Autodesk Fusion 360 part; units mm, degrees
note: some values were not read from the file. Chosen so that the rebuilt part matches the saved one: which bodies a step acts on. Set by a fixed rule: which sketch regions a step uses.
(part 2 of 2)
sketch "Sketch33" plane through (0, 0, 0.2628) normal (0, 0, -1) x (1, 0, 0)
  circle A0 centre (90.2873, -26.9645) radius 2.5
  circle A1 centre (90.2873, -69.9645) radius 2.5
  line L0 (125, -25) -> (125, 0)
  line L1 (125, 0) -> (70.3336, 0)
  line L2 (70.3336, 0) -> (70.3336, -89.9645)
  line L3 (70.3336, -89.9645) -> (220.2873, -89.9645)
  line L4 (220.2873, -89.9645) -> (220.2873, 0.0355)
  line L5 (220.2873, 0.0355) -> (200.2873, 0.0355)
  line L6 (200.2873, 0.0355) -> (200.2873, 0)
  line L7 (200.2873, 0) -> (150.3104, 0)
  line L8 (150.3104, 0) -> (150.3104, -25)
  line L9 (150.3104, -25) -> (125, -25)
  circle A2 centre (136.2, -48.4645) radius 2
  circle A3 centre (200.2873, -69.9645) radius 2.5
  circle A4 centre (200.2873, -26.9645) radius 2.5
  line L10 (125, -25) -> (105, -25)
  line L11 (105, -25) -> (105, 0)
  constraint coincident L0.start L9.end
  constraint perpendicular L0 L10
  constraint perpendicular L9 L11
extrude "Extrude49" cut sketch "Sketch33" against normal blind 18 contours L0 L1 L10 L11 bodies 4
sketch "Sketch34" plane through (0, 0, 0) normal (0, 0, 1) x (1, 0, 0)
sketch "Sketch35" plane through (0, 0, -47.7372) normal (0, 0, -1) x (1, 0, 0)
  line L0 (142.4, -37.0645) -> (142.4, -59.8645)
  line L1 (142.4, -59.8645) -> (130, -59.8645)
  line L2 (130, -59.8645) -> (130, -37.0645)
  line L3 (130, -37.0645) -> (142.4, -37.0645)
  circle A0 centre (136.2, -62.8645) radius 1.5
  circle A1 centre (136.2, -34.0645) radius 1.5
  line L4 (146.4, -29.0645) -> (126, -29.0645)
  line L5 (126, -29.0645) -> (126, -67.8645)
  line L6 (126, -67.8645) -> (146.4, -67.8645)
  line L7 (146.4, -67.8645) -> (146.4, -29.0645)
  line L8 (-49.6, -20) -> (-49.6, -58.8)
  line L9 (-49.6, -58.8) -> (-70, -58.8)
  line L10 (-70, -58.8) -> (-70, -20)
  line L11 (-53.6, -50.8) -> (-66, -50.8)
  line L12 (-53.6, -44) -> (-53.6, -50.8)
  line L13 (-66, -44) -> (-66, -50.8)
  line L14 (-59.8, -41) -> (-56.3, -41)
  line L15 (-59.8, -41) -> (-63.3, -41)
  line L16 (-56.3, -19) -> (-63.3, -19)
  line L17 (-63.3, -19) -> (-63.3, -41)
  line L18 (-70, -20) -> (-66.3, -20)
  line L19 (-53.3, -20) -> (-49.6, -20)
  line L20 (-63.3, -19) -> (-63.3, -20)
  line L21 (-53.3, -19) -> (-53.3, -16)
  line L22 (-53.3, -16) -> (-53.3, -20)
  line L23 (-53.3, -16) -> (-67, -16)
  line L24 (-66.3, -19) -> (-66.3, -16)
  line L25 (-66.3, -19) -> (-66.3, -44)
  line L26 (-66.3, -44) -> (-53.3, -44)
  line L27 (-53.3, -20) -> (-53.3, -44)
  line L28 (-56.3, -19) -> (-56.3, -41)
  dimension "d215" = 20.4
  dimension "d216" = 38.8
  dimension "d224" = 3.5
  dimension "d225" = 3.5
  dimension "d226" = 22
  dimension "d227" = 7
  dimension "d228" = 3
  dimension "d229" = 3
  dimension "d230" = 3
  constraint horizontal L18
  constraint vertical L8
  constraint horizontal L9
  constraint vertical L10
  constraint perpendicular L10 L11
  constraint perpendicular L11 L12
  constraint perpendicular L11 L13
  constraint coincident L17 L20.end
  constraint collinear L18 L19
  constraint perpendicular L16 L20
  constraint parallel L12 L22
  constraint perpendicular L21 L23
  constraint coincident L23 L24.end
  constraint perpendicular L23 L24
  constraint perpendicular L22 L26
  constraint coincident L25 L18.end
  constraint coincident L26 L13.start
  constraint coincident L26 L12.start
  constraint perpendicular L26 L27
  constraint perpendicular L14 L28
  measures "d215" distance of L10.end L8.start
  measures "d216" distance of L10.end L9.end
  measures "d224" distance of L14.start L14.end
  measures "d225" distance of L14.start L15.end
  measures "d226" distance of L14.end L16.start
  measures "d227" distance of L16.start L16.end
  measures "d228" distance of L16.end L24.start
  measures "d229" distance of L16.start L21.start
  measures "d230" distance of L21.start L21.end
extrude "Extrude50" add sketch "Sketch35" along normal blind 7 separate body contours L21 L22 L23 L24 L25 L26 L27 makes body 5
sketch "Sketch36" plane through (0, 0, -54.7372) normal (0, 0, -1) x (1, 0, 0)
  line L0 (-63.3, -41) -> (-63.3, -19)
  line L1 (-63.3, -19) -> (-56.3, -19)
  line L2 (-56.3, -19) -> (-56.3, -41)
  line L3 (-56.3, -41) -> (-63.3, -41)
  line L4 (-53.3, -16) -> (-66.3, -16)
  line L5 (-66.3, -16) -> (-66.3, -44)
  line L6 (-66.3, -44) -> (-53.3, -44)
  line L7 (-53.3, -44) -> (-53.3, -16)
  line L8 (-66.3, -16) -> (-53.3, -16)
  line L9 (-53.3, -16) -> (-46.8, -16)
  line L10 (-66.3, -16) -> (-72.8, -16)
  line L11 (-72.8, -16) -> (-77.8, -16)
  line L12 (-46.8, -16) -> (-41.8, -16)
  line L13 (-46.8, -16) -> (-46.8, -44)
  line L14 (-46.8, -44) -> (-46.8, -49)
  line L15 (-72.8, -16) -> (-72.8, -44)
  line L16 (-72.8, -44) -> (-72.8, -49)
  line L17 (-72.8, -49) -> (-46.8, -49)
  line L18 (-72.8, -16) -> (-72.8, -11)
  line L19 (-72.8, -11) -> (-47, -11)
  line L20 (-47, -11) -> (-42, -11)
  line L21 (-42, -11) -> (-42, -49)
  line L22 (-42, -49) -> (-46.8, -49)
  line L23 (-72.8, -49) -> (-77.8, -49)
  line L24 (-77.8, -49) -> (-77.8, -11)
  line L25 (-77.8, -11) -> (-72.8, -11)
  line L26 (-77.8, -11) -> (-77.8, -6)
  line L27 (-42, -11) -> (-42, -6)
  dimension "d233" = 6.5
  dimension "d234" = 6.5
  dimension "d235" = 5
  dimension "d236" = 5
  dimension "d237" = 5
  dimension "d238" = 5
  dimension "d239" = 5
  dimension "d240" = 5
  dimension "d241" = 5
  dimension "d242" = 5
  constraint coincident L4.end L5.start
  constraint coincident L4.start L7.end
  constraint perpendicular L7 L9
  constraint perpendicular L5 L10
  constraint perpendicular L0 L11
  constraint perpendicular L7 L12
  constraint perpendicular L9 L13
  constraint perpendicular L9 L14
  constraint perpendicular L11 L15
  constraint perpendicular L11 L16
  constraint perpendicular L14 L17
  constraint perpendicular L10 L18
  constraint perpendicular L18 L19
  constraint perpendicular L18 L20
  constraint perpendicular L20 L21
  constraint perpendicular L16 L23
  constraint perpendicular L11 L24
  constraint perpendicular L25 L26
  constraint perpendicular L20 L27
  measures "d233" distance of L4.start L9.end
  measures "d234" distance of L4.end L10.end
  measures "d235" distance of L10.end L11.end
  measures "d236" distance of L9.end L12.end
  measures "d237" distance of L13.end L14.end
  measures "d238" distance of L15.end L16.end
  measures "d239" distance of L10.end L18.end
  measures "d240" distance of L16.end L23.end
  measures "d241" distance of L24.end L26.end
  measures "d242" distance of L20.end L27.end
extrude "Extrude51" add sketch "Sketch36" along normal blind 5 contours L0 L1 L2 L3 | L4 L5 L6 L7 L8 | L5 L6 L7 L9 L10 L13 L14 L15 L16 L17 | L4 L8 L9 L10 L12 L18 L19 L20 L21 | L12 L13 L14 L21 L22 | L11 L15 L16 L23 L24 | L11 L18 L24 L25 bodies 5
extrude "Extrude52" cut 1 faces at (-65.8, 36.3333, -59.7372) along direction (0, 0, 1) blind 2 on bodies 5 bodies 5
sketch "Sketch37" plane through (0, 0, -57.7372) normal (0, 0, -1) x (1, 0, 0)
  line L0 (-77.8, -49) -> (-46.8, -49)
  line L1 (-46.8, -49) -> (-42, -49)
  line L2 (-42, -49) -> (-42, -11)
  line L3 (-42, -11) -> (-72.8, -11)
  line L4 (-72.8, -11) -> (-77.8, -11)
  line L5 (-77.8, -11) -> (-77.8, -49)
  line L6 (-77.8, -11) -> (-72.8, -11)
  line L7 (-72.8, -11) -> (-72.8, -49)
  line L8 (-42, -11) -> (-47, -11)
  line L9 (-47, -11) -> (-46.8, -49)
  dimension "d247" = 5
  dimension "d248" = 5
  constraint coincident L4.end L5.start
  constraint perpendicular L5 L6
  constraint coincident L0 L7.end
  constraint perpendicular L0 L7
  constraint coincident L2.end L3.start
  constraint perpendicular L2 L8
  constraint coincident L0.end L1.start
  measures "d247" distance of L4.end L3.end
  measures "d248" distance of L2.end L8.end
extrude "Extrude53" add sketch "Sketch37" along normal blind 30 contours L0 L4 L5 L6 L7 | L1 L2 L3 L8 L9 bodies 5
sketch "Sketch38" plane through (0, 0, -57.7372) normal (0, 0, -1) x (1, 0, 0)
  line L0 (-46.8, -49) -> (-47, -11)
  line L1 (-47, -11) -> (-72.8, -11)
  line L2 (-72.8, -11) -> (-72.8, -49)
  line L3 (-72.8, -49) -> (-46.8, -49)
  line L4 (-59.9, -11) -> (-59.9, -16)
  line L5 (-59.9, -16) -> (-72.8, -16)
  line L6 (-59.9, -16) -> (-46.974, -15.932)
  dimension "d251" = 5
  constraint midpoint L1 L4.start
  constraint perpendicular L1 L4
  constraint coincident L2 L5.end
  constraint perpendicular L2 L5
  constraint coincident L0 L6.end
  constraint perpendicular L0 L6
  measures "d251" distance of L4.start L4.end
extrude "Extrude54" add sketch "Sketch38" along normal blind 30 contours L0 L1 L4 L6 | L1 L2 L4 L5 bodies 5
sketch "Sketch39" plane through (0, 0, -57.7372) normal (0, 0, -1) x (1, 0, 0)
  line L0 (-59.9, -16) -> (-72.8, -16)
  line L1 (-72.8, -16) -> (-72.8, -49)
  line L2 (-72.8, -49) -> (-46.8, -49)
  line L3 (-46.8, -49) -> (-46.974, -15.932)
  line L4 (-46.974, -15.932) -> (-59.9, -16)
extrude "Extrude55" add 1 faces at (-77.8, 36.3333, -65.7372) along direction (-1, 0, 0) blind 2.5 on bodies 5 bodies 5
extrude "Extrude56" cut 1 faces at (-72.8, 27, -77.7372) along direction (-1, 0, 0) blind 2.5 on bodies 5 bodies 5
extrude "Extrude57" add 1 faces at (-42, 36.3333, -65.7372) along direction (1, 0, 0) blind 2.5 on bodies 5 bodies 5
extrude "Extrude58" cut 1 faces at (-46.916, 26.9546, -77.7372) along direction (0.999986, -0.005263, 0) blind 2.5 on bodies 5 bodies 5
delete_face "DeleteFace1" 1 faces at (-43.6, 49, -66.7372) on bodies 5
extrude "Extrude59" add 1 faces at (-45.9667, 48.9956, -77.7372) along direction (-0.005263, -0.999986, 0) blind 5 on bodies 5 bodies 5
sketch "Sketch40" plane through (0, 0, -87.7372) normal (0, 0, -1) x (1, 0, 0)
  line L0 (-46.8, -49) -> (-39.5, -49)
  line L1 (-39.5, -49) -> (-39.5, -11)
  line L2 (-39.5, -11) -> (-80.3, -11)
  line L3 (-80.3, -11) -> (-80.3, -49)
  line L4 (-80.3, -49) -> (-75.3, -49)
  line L5 (-75.3, -49) -> (-75.3, -16)
  line L6 (-75.3, -16) -> (-59.9, -16)
  line L7 (-59.9, -16) -> (-44.4741, -15.9188)
  line L8 (-44.4741, -15.9188) -> (-44.3264, -43.9869)
  line L9 (-44.3264, -43.9869) -> (-46.8263, -44.0001)
  line L10 (-46.8263, -44.0001) -> (-46.8, -49)
  line L11 (-44.3264, -43.9869) -> (-44.3264, -49)
  constraint coincident L8.end L9.start
  constraint coincident L0 L11.end
  constraint perpendicular L0 L11
extrude "Extrude60" cut sketch "Sketch40" against normal blind 30 contours L0 L9 L10 L11 bodies 5
sketch "Sketch41" plane through (0, 0, -6.7372) normal (0, 0, -1) x (1, 0, 0)
  circle A0 centre (136.2, -48.4645) radius 2
  line L0 (142.4, -59.3645) -> (146.4, -59.3645)
  line L1 (146.4, -59.3645) -> (146.4, -37.3645)
  line L2 (146.4, -37.3645) -> (142.4, -37.3645)
  line L3 (142.4, -37.3645) -> (142.4, -37.0645)
  line L4 (142.4, -37.0645) -> (130, -37.0645)
  line L5 (130, -37.0645) -> (130, -37.3645)
  line L6 (130, -37.3645) -> (126, -37.3645)
  line L7 (126, -37.3645) -> (126, -59.3645)
  line L8 (126, -59.3645) -> (130, -59.3645)
  line L9 (130, -59.3645) -> (130, -59.8645)
  line L10 (130, -59.8645) -> (142.4, -59.8645)
  line L11 (142.4, -59.8645) -> (142.4, -59.3645)
  line L12 (136.2, -48.4645) -> (136.2, -25)
  line L13 (136.2, -25) -> (136.2, -31)
  line L14 (136.2, -25) -> (136.2, -31)
  line L15 (136.2, -31) -> (136.2, -15)
  line L16 (136.2, -15) -> (136.2, -12)
  line L17 (136.2, -12) -> (146, -12)
  line L18 (146, -12) -> (128, -12)
  dimension "d266" = 6
  dimension "d267" = 6
  dimension "d268" = 16
  dimension "d269" = 3
  constraint coincident A0.centre L12.start
  constraint perpendicular L4 L12
  constraint perpendicular L4 L13
  constraint perpendicular L4 L14
  constraint parallel L12 L15
  constraint parallel L15 L16
  constraint perpendicular L16 L17
  constraint parallel L17 L18
  measures "d266" distance of L12.end L13.end
  measures "d267" distance of L12.end L13.end
  measures "d268" distance of L13.end L15.end
  measures "d269" distance of L15.end L16.end
sketch "Sketch42" plane through (0, 0, -54.7372) normal (0, 0, 1) x (-1, 0, 0)
  line L0 (53.3, -44) -> (53.3, -16)
  line L1 (53.3, -16) -> (66.3, -16)
  line L2 (66.3, -16) -> (66.3, -44)
  line L3 (66.3, -44) -> (53.3, -44)
  line L4 (39.5, -49) -> (80.3, -49)
  line L5 (80.3, -49) -> (80.3, -11)
  line L6 (80.3, -11) -> (77.8, -11)
  line L7 (77.8, -11) -> (72.8, -11)
  line L8 (72.8, -11) -> (39.5, -11)
  line L9 (39.5, -11) -> (39.5, -49)
sketch "Sketch43" plane through (0, 0, -57.7372) normal (0, 0, -1) x (1, 0, 0)
  line L0 (-60, -49) -> (-60, -44)
  dimension "d270" = 5
  constraint vertical L0
  measures "d270" distance of L0.start L0.end
sketch "Sketch44" plane through (0, 49, 0) normal (0, 1, 0) x (-1, 0, 0)
  line L0 (44.3264, -57.7372) -> (75.3, -57.7372)
  line L1 (75.3, -57.7372) -> (75.3, -87.7372)
  line L2 (75.3, -87.7372) -> (80.3, -87.7372)
  line L3 (80.3, -87.7372) -> (80.3, -54.7372)
  line L4 (80.3, -54.7372) -> (39.5, -54.7372)
  line L5 (39.5, -54.7372) -> (39.5, -87.7372)
  line L6 (39.5, -87.7372) -> (44.3264, -87.7372)
  line L7 (44.3264, -87.7372) -> (44.3264, -57.7372)
extrude "Extrude61" add sketch "Sketch44" along normal blind 8 bodies 5
extrude "Extrude62" cut 1 faces at (-78.6333, 57, -66.7372) along direction (0, -1, 0) blind 13 on bodies 5 bodies 5
sketch "Sketch45" plane through (0, 44, 0) normal (0, 1, 0) x (-1, 0, 0)
  line L0 (66.3, -47.7372) -> (53.3, -47.7372)
  line L1 (53.3, -47.7372) -> (53.3, -54.7372)
  line L2 (53.3, -54.7372) -> (39.5, -54.7372)
  line L3 (39.5, -54.7372) -> (39.5, -87.7372)
  line L4 (39.5, -87.7372) -> (44.3264, -87.7372)
  line L5 (44.3264, -87.7372) -> (44.3264, -57.7372)
  line L6 (44.3264, -57.7372) -> (75.3, -57.7372)
  line L7 (75.3, -57.7372) -> (75.3, -87.7372)
  line L8 (75.3, -87.7372) -> (80.3, -87.7372)
  line L9 (80.3, -87.7372) -> (80.3, -54.7372)
  line L10 (80.3, -54.7372) -> (66.3, -54.7372)
  line L11 (66.3, -54.7372) -> (66.3, -47.7372)
  line L12 (44.3264, -57.7372) -> (44.3264, -54.7372)
  line L13 (75.3, -57.7372) -> (75.3, -54.7372)
  constraint coincident L5.end L6.start
  constraint coincident L2 L12.end
  constraint perpendicular L2 L12
  constraint coincident L6.end L7.start
  constraint coincident L10 L13.end
  constraint perpendicular L10 L13
extrude "Extrude63" add sketch "Sketch45" along normal blind 30 contours L7 L8 L9 L10 L13 | L2 L3 L4 L5 L12 bodies 5
extrude "Extrude64" add 2 faces at (-41.1088, 74, -65.7372) (-76.9667, 74, -65.7372) along direction (0, 1, 0) blind 10 on bodies 5 bodies 5
extrude "Extrude65" add 1 faces at (-59.8421, 34.6623, -57.7372) along direction (0, 0, -1) blind 30 on bodies 5 bodies 5
extrude "Extrude66" add 2 faces at (-41.1088, 84, -65.7372) (-76.9667, 84, -65.7372) along direction (0, 1, 0) blind 5 on bodies 5 bodies 5
sketch "Sketch46" plane through (-80.3, 0, 0) normal (-1, 0, 0) x (0, -1, 0)
  line L0 (-89, -87.7372) -> (-11, -87.7372)
  line L1 (-11, -87.7372) -> (-11, -54.7372)
  line L2 (-11, -54.7372) -> (-89, -54.7372)
  line L3 (-89, -54.7372) -> (-89, -87.7372)
  line L4 (-89, -65.3059) -> (-81, -65.3059)
  line L5 (-89, -54.7372) -> (-89, -62.7372)
  line L6 (-89, -62.7372) -> (-81, -62.7372)
  line L7 (-81, -62.7372) -> (-81, -57.7372)
  line L8 (-81, -65.3059) -> (-64, -65.3059)
  line L9 (-81, -62.7372) -> (-64, -62.7372)
  line L10 (-81, -65.3059) -> (-81, -57.3059)
  line L11 (-81, -57.3059) -> (-64, -57.3059)
  line L12 (-64, -57.3059) -> (-64, -65.3059)
  dimension "d283" = 8
  dimension "d284" = 8
  dimension "d285" = 8
  dimension "d286" = 5
  dimension "d287" = 17
  dimension "d288" = 17
  dimension "d289" = 8
  constraint coincident L3 L4.start
  constraint perpendicular L3 L4
  constraint coincident L2.end L3.start
  constraint perpendicular L4 L5
  constraint perpendicular L5 L6
  constraint perpendicular L4 L7
  constraint perpendicular L3 L8
  constraint perpendicular L7 L9
  constraint perpendicular L6 L10
  constraint perpendicular L10 L11
  measures "d283" distance of L4.start L4.end
  measures "d284" distance of L2.end L5.end
  measures "d285" distance of L5.end L6.end
  measures "d286" distance of L6.end L7.end
  measures "d287" distance of L4.end L8.end
  measures "d288" distance of L6.end L9.end
  measures "d289" distance of L4.end L10.end
extrude "Extrude67" add sketch "Sketch46" along normal blind 13 contours L8 L9 L10 L12 | L7 L9 L10 L11 L12 bodies 5
sketch "Sketch47" plane through (0, 81, 0) normal (0, 1, 0) x (-1, 0, 0)
  line L0 (80.3, -57.3059) -> (80.3, -65.3059)
  line L1 (80.3, -65.3059) -> (93.3, -65.3059)
  line L2 (93.3, -65.3059) -> (93.3, -57.3059)
  line L3 (93.3, -57.3059) -> (80.3, -57.3059)
  line L4 (80.3, -65.3059) -> (86.3, -65.3059)
  line L5 (86.3, -65.3059) -> (86.3, -62.3059)
  circle A0 centre (86.3, -62.3059) radius 1.5
  dimension "d292" = 6
  dimension "d293" = 3
  dimension "d294" = 3
  constraint coincident L0.end L1.start
  constraint perpendicular L0 L4
  constraint perpendicular L4 L5
  constraint coincident L5.end A0.centre
  measures "d292" distance of L0.end L4.end
  measures "d293" distance of L4.end L5.end
  measures "d294" diameter of A0
extrude "Extrude68" cut sketch "Sketch47" against normal blind 13 contours A0 bodies 5
extrude "Extrude69" cut 1 faces at (-88.9667, 75.3333, -57.3059) along direction (0, 0, -1) blind 2 on bodies 5 bodies 5
extrude "Extrude70" add 1 faces at (-52.2088, 22, -87.7372) along direction (0, 0, -1) blind 5 on bodies 5 bodies 5
sketch "Sketch48" plane through (0, 89, 0) normal (0, 1, 0) x (-1, 0, 0)
  line L0 (80.3, -92.7372) -> (80.3, -54.7372)
  line L1 (80.3, -54.7372) -> (75.3, -54.7372)
  line L2 (75.3, -54.7372) -> (75.3, -92.7372)
  line L3 (75.3, -92.7372) -> (80.3, -92.7372)
sketch "Sketch49" plane through (-80.3, 0, 0) normal (-1, 0, 0) x (0, -1, 0)
  line L0 (-81, -65.3059) -> (-81, -59.3059)
  line L1 (-81, -59.3059) -> (-64, -59.3059)
  line L2 (-64, -59.3059) -> (-64, -65.3059)
  line L3 (-64, -65.3059) -> (-81, -65.3059)
  line L4 (-11, -92.7372) -> (-11, -54.7372)
  line L5 (-11, -54.7372) -> (-89, -54.7372)
  line L6 (-89, -54.7372) -> (-89, -92.7372)
  line L7 (-89, -92.7372) -> (-11, -92.7372)
sketch "Sketch50" plane through (0, 89, 0) normal (0, 1, 0) x (-1, 0, 0)
sketch "Sketch51" plane through (-80.3, 0, 0) normal (-1, 0, 0) x (0, -1, 0)
sketch "Sketch52" plane through (0, 0, 0) normal (0, 1, 0) x (1, 0, 0)
  line L0 (-10, -20) -> (-50.8, -20)
  line L1 (-50.8, -20) -> (-50.8, -58)
  line L2 (-50.8, -58) -> (-50.8, -49)
  line L3 (-53.3, -49) -> (-56.8, -49)
  line L4 (-56.8, -49) -> (-60.3, -49)
  line L5 (-56.8, -49) -> (-53.3, -49)
  line L6 (-56.8, -49) -> (-60.3, -49)
  line L7 (-53.3, -49) -> (-53.3, -65)
  line L8 (-60.3, -49) -> (-60.3, -65)
  line L9 (-60.3, -65) -> (-53.3, -65)
  line L10 (-82, -49) -> (-82, -46)
  line L11 (-63.3, -46) -> (-50.8, -46)
  line L12 (-63.3, -68) -> (-50.8, -68)
  line L13 (-50.8, -68) -> (-50.8, -58)
  line L14 (-72.8, 54.7372) -> (-39.5, 54.7372)
  line L15 (-39.5, 92.7372) -> (-80.3, 92.7372)
  line L16 (-60.3, -49) -> (-63.3, -49)
  line L17 (-63.3, -49) -> (-63.3, -68)
  line L18 (-63.3, -49) -> (-63.3, -46)
  line L19 (-50.8, -68) -> (-10, -68)
  line L20 (-10, -20) -> (-10, -68)
  dimension "d301" = 38
  dimension "d302" = 9
  dimension "d303" = 6
  dimension "d305" = 3.5
  dimension "d306" = 3.5
  dimension "d307" = 16
  dimension "d308" = 16
  dimension "d311" = 3
  dimension "d312" = 33.3
  dimension "d313" = 40.8
  dimension "d314" = 40.8
  dimension "d315" = 3
  constraint horizontal L0
  constraint perpendicular L0 L1
  constraint parallel L1 L2
  constraint perpendicular L2 L3
  constraint parallel L3 L4
  constraint parallel L3 L5
  constraint perpendicular L2 L6
  constraint perpendicular L5 L7
  constraint perpendicular L4 L8
  constraint coincident L1 L11.end
  constraint perpendicular L1 L11
  constraint perpendicular L9 L13
  constraint perpendicular L8 L16
  constraint perpendicular L12 L17
  constraint perpendicular L11 L18
  constraint perpendicular L13 L19
  constraint perpendicular L19 L20
  measures "d301" distance of L0.end L1.end
  measures "d302" distance of L1.end L2.end
  measures "d303" distance of L2.end L3.end
  measures "d305" distance of L3.end L3.start
  measures "d306" distance of L3.end L4.end
  measures "d307" distance of L3.start L7.end
  measures "d308" distance of L4.end L8.end
  measures "d311" distance of L10.start L10.end
  measures "d312" distance of L14.start L14.end
  measures "d313" distance of L15.start L15.end
  measures "d314" distance of L0.start L0.end
  measures "d315" distance of L4.end L16.end
extrude "Extrude71" add sketch "Sketch52" along normal blind 5 separate body makes body 6
sketch "Sketch53" plane through (0, 5, 0) normal (0, 1, 0) x (-1, 0, 0)
  line L0 (60.3, 49) -> (53.3, 49)
  line L1 (53.3, 49) -> (53.3, 65)
  line L2 (53.3, 65) -> (60.3, 65)
  line L3 (60.3, 65) -> (60.3, 49)
  line L4 (50.8, 20) -> (50.8, 46)
  line L5 (50.8, 46) -> (63.3, 46)
  line L6 (63.3, 46) -> (63.3, 68)
  line L7 (63.3, 68) -> (10, 68)
  line L8 (10, 68) -> (10, 20)
  line L9 (10, 20) -> (50.8, 20)
  line L10 (53.3, 65) -> (60.3, 65)
  line L11 (60.3, 65) -> (60.3, 49)
  line L12 (60.3, 49) -> (53.3, 49)
  line L13 (53.3, 49) -> (53.3, 65)
  constraint horizontal L10
  constraint vertical L11
  constraint horizontal L12
  constraint vertical L13
  constraint coincident L0.start L3.end
  constraint coincident L1.end L2.start
extrude "Extrude72" add sketch "Sketch53" against normal blind 2 contours L0 L1 L2 L3 L10 L11 L12 L13 bodies 6
move_body "Move3" bodies 6 to x (1, 0, 0) y (0, 1, 0) z (0, 0, 1) at (-31.7357, 93.4456, -113.0049)
sketch "Sketch54" plane through (150.2873, 0, 0) normal (-1, 0, 0) x (0, -1, 0)
  line L0 (-25, 7.2628) -> (-25, 18.2628)
  line L1 (-25, 18.2628) -> (-21.9645, 18.2628)
  line L2 (-21.9645, 18.2628) -> (-21.9645, 50.4628)
  line L3 (-21.9645, 50.4628) -> (-69.9645, 50.4628)
  line L4 (-69.9645, 50.4628) -> (-69.9645, 7.2628)
  line L5 (-69.9645, 7.2628) -> (-25, 7.2628)
  circle A0 centre (-64.3645, 12.8628) radius 1.5
  circle A1 centre (-64.3645, 44.8628) radius 1.5
  circle A2 centre (-32.5645, 12.8628) radius 1.5
  circle A3 centre (-32.5645, 44.8628) radius 1.5
  circle A4 centre (-48.4645, 28.8628) radius 11.5
  line L6 (-48.4645, 28.8628) -> (-21.9645, 28.8628)
  constraint coincident A4.centre L6.start
  constraint coincident L2 L6.end
  constraint perpendicular L2 L6
sketch "Sketch55" plane through (150.2873, 0, 0) normal (-1, 0, 0) x (0, -1, 0)
  line L0 (-150, 30) -> (-180, 30)
  line L1 (-180, 30) -> (-180, 35)
  line L2 (-180, 30) -> (-180, 25)
  line L3 (-180, 35) -> (-150, 35)
  line L4 (-150, 35) -> (-150, 25)
  line L5 (-150, 25) -> (-180, 25)
  line L6 (-150, 35) -> (-140, 35)
  line L7 (-140, 35) -> (-140, -65)
  line L8 (-150, 25) -> (-150, -65)
  line L9 (-150, -65) -> (-140, -65)
  dimension "d320" = 30
  dimension "d321" = 5
  dimension "d322" = 5
  dimension "d323" = 10
  dimension "d324" = 100
  dimension "d325" = 90
  constraint horizontal L0
  constraint perpendicular L0 L1
  constraint perpendicular L0 L2
  constraint perpendicular L1 L3
  constraint perpendicular L0 L4
  constraint perpendicular L2 L5
  constraint perpendicular L4 L6
  constraint perpendicular L6 L7
  constraint perpendicular L5 L8
  measures "d320" distance of L0.start L0.end
  measures "d321" distance of L0.end L1.end
  measures "d322" distance of L0.end L2.end
  measures "d323" distance of L3.end L6.end
  measures "d324" distance of L6.end L7.end
  measures "d325" distance of L4.end L8.end
extrude "Extrude73" add sketch "Sketch55" along normal blind 10 separate body makes body 7
sketch "Sketch56" plane through (0, 0, -65) normal (0, 0, -1) x (1, 0, 0)
  line L0 (150.2873, -150) -> (150.2873, -140)
  line L1 (150.2873, -140) -> (140.2873, -140)
  line L2 (140.2873, -140) -> (140.2873, -150)
  line L3 (140.2873, -150) -> (150.2873, -150)
  line L4 (140.2873, -150) -> (145.2873, -150)
  line L5 (145.2873, -150) -> (145.2873, -145)
  circle A0 centre (145.2873, -145) radius 5
  dimension "d328" = 5
  dimension "d329" = 5
  dimension "d330" = 10
  constraint coincident L2.end L3.start
  constraint perpendicular L2 L4
  constraint perpendicular L4 L5
  constraint coincident L5.end A0.centre
  measures "d328" distance of L2.end L4.end
  measures "d329" distance of L4.end L5.end
  measures "d330" diameter of A0
extrude "Extrude74" cut sketch "Sketch56" against normal blind 90 contours L0 L3 A0 | L0 L1 A0 | L2 L3 L4 A0 | L1 L2 A0 bodies 7
extrude "Extrude75" add 1 faces at (146.954, 180, 31.6667) along direction (0, 1, 0) blind 8 on bodies 7 bodies 7
sketch "Sketch57" plane through (140.2873, 0, 0) normal (-1, 0, 0) x (0, -1, 0)
  line L0 (-188, 25) -> (-145, 25)
  line L1 (-145, 25) -> (-140, 25)
  line L2 (-140, 25) -> (-140, 35)
  line L3 (-140, 35) -> (-188, 35)
  line L4 (-188, 35) -> (-188, 25)
  line L5 (-188, 30) -> (-182.5, 30)
  circle A0 centre (-182.5, 30) radius 2.5
  circle A1 centre (-182.5, 30) radius 5
  dimension "d335" = 5.5
  dimension "d336" = 5
  dimension "d337" = 10
  constraint midpoint L4 L5.start
  constraint perpendicular L4 L5
  constraint coincident L5.end A0.centre
  constraint concentric A0 A1
  measures "d335" distance of L5.start L5.end
  measures "d336" diameter of A0
  measures "d337" diameter of A1
extrude "Extrude76" add sketch "Sketch57" along normal blind 10 contours A1 bodies 7
extrude "Extrude77" cut 1 faces at (140.2873, 181.5231, 29.169) along direction (1, 0, 0) blind 10 on bodies 7 bodies 7
extrude "Extrude78" add 1 faces at (130.2873, 185.7097, 32.6393) along direction (-1, 0, 0) blind 10 on bodies 7 bodies 7
sketch "Sketch58" plane through (0, 188, 0) normal (0, 1, 0) x (-1, 0, 0)
  line L0 (-150.2873, 35) -> (-150.2873, 25)
  line L1 (-150.2873, 25) -> (-140.2873, 25)
  line L2 (-140.2873, 25) -> (-140.2873, 35)
  line L3 (-140.2873, 35) -> (-150.2873, 35)
  line L4 (-140.2873, 35) -> (-120, 35)
  line L5 (-140.2873, 25) -> (-120, 25)
  line L6 (-120, 35) -> (-120, 25)
  constraint coincident L2.end L3.start
  constraint perpendicular L2 L4
  constraint coincident L1.end L2.start
  constraint perpendicular L2 L5
  constraint perpendicular L5 L6
extrude "Extrude79" cut sketch "Sketch58" against normal blind 2 contours L2 L4 L5 L6 bodies 7
sketch "Sketch59" plane through (0, 188, 0) normal (0, 1, 0) x (-1, 0, 0)
  line L0 (-150.2873, 35) -> (-150.2873, 25)
  line L1 (-150.2873, 25) -> (-140.2873, 25)
  line L2 (-140.2873, 25) -> (-140.2873, 35)
  line L3 (-140.2873, 35) -> (-150.2873, 35)
  line L4 (-140.2873, 35) -> (-120, 35)
  line L5 (-140.2873, 25) -> (-120, 25)
  line L6 (-120, 25) -> (-120, 35)
  constraint coincident L2.end L3.start
  constraint perpendicular L2 L4
  constraint coincident L1.end L2.start
  constraint perpendicular L2 L5
  constraint perpendicular L4 L6
extrude "Extrude80" add sketch "Sketch59" against normal blind 2 contours L2 L4 L5 L6 bodies 7
sketch "Sketch60" plane through (0, 188, 0) normal (0, 1, 0) x (-1, 0, 0)
  line L0 (-150.2873, 35) -> (-150.2873, 25)
  line L1 (-150.2873, 25) -> (-120, 25)
  line L2 (-120, 25) -> (-120, 35)
  line L3 (-120, 35) -> (-150.2873, 35)
  line L4 (-130, 25) -> (-130, 30)
  circle A0 centre (-130, 30) radius 2
  dimension "d348" = 4
  constraint coincident L1 L4.start
  constraint perpendicular L1 L4
  constraint coincident L4.end A0.centre
  measures "d348" diameter of A0
extrude "Extrude81" cut sketch "Sketch60" against normal blind 5 contours A0 bodies 7
extrude "Extrude82" cut 1 faces at (143.9102, 145.9389, -65) along direction (0, 0, 1) blind 100 on bodies 7 bodies 7
sketch "Sketch61" plane through (0, 0, 25) normal (0, 0, -1) x (1, 0, 0)
  line L0 (150.2873, -188) -> (150.2873, -145)
  arc A0 (140.2873, -145) -> (150.2873, -145) centre (145.2873, -145) ccw
  line L1 (140.2873, -145) -> (140.2873, -182.5)
  line L2 (140.2873, -182.5) -> (140.2873, -186)
  line L3 (140.2873, -186) -> (120, -186)
  line L4 (120, -186) -> (120, -188)
  line L5 (120, -188) -> (150.2873, -188)
  circle A1 centre (145.2873, -145) radius 5
  constraint concentric A0 A1
  constraint coincident A0.start A1
extrude "Extrude83" add sketch "Sketch61" against normal blind 100 contours A0 A1 bodies 7
move_body "Move4" bodies 7 to x (-0.996195, -0.087156, 0) y (-0.087156, 0.996195, 0) z (0, 0, -1) at (-953.1386, -95.4596, 367.2047)
move_body "Move5" bodies 7 to x (1, 0, 0) y (0, 1, 0) z (0, 0, 1) at (1242.5842, -19.7779, -319.8037)
move_body "Move6" bodies 7 to x (1, 0, 0) y (0, 1, 0) z (0, 0, 1) at (0, -10, 10)
move_body "Move7" bodies 7 to x (1, 0, 0) y (0, 1, 0) z (0, 0, 1) at (-19.9239, 0, 1.7431)
move_body "Move8" bodies 5 to x (1, 0, 0) y (0, 1, 0) z (0, 0, 1) at (81.9371, 11.3602, -17.2934)
extrude "Extrude84" add 1 faces at (115.8401, 7.1203, -65.8559) along direction (0, 0, -1) blind 28 on bodies 7 bodies 7
extrude "Extrude85" cut 1 faces at (115.8401, 7.1203, -93.8559) along direction (0, 0, 1) blind 5 on bodies 7 bodies 7
extrude "Extrude86" add 1 faces at (115.8401, 7.1203, -88.8559) along direction (0, 0, -1) blind 3 on bodies 7 bodies 7
move_body "Move9" bodies 5 to x (1, 0, 0) y (0, 1, 0) z (0, 0, 1) at (-86.3589, 8.941, 19.1613)
move_body "Move10" bodies 5 to x (1, 0, 0) y (0, 1, 0) z (0, 0, 1) at (-9.9033, -18.9, 4.6405)
hidden bodies 2 7
